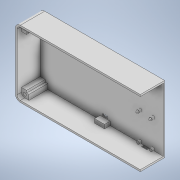
# Autodesk Inventor part: Case Left Half
Saved by Autodesk Inventor 2020 (Build 240168000, 168)
## iProperties
Created: 2021-04-14
Part Number: Case Left Half
Material: Generic
Document SubType Name: Modeling
Designer: user
Density: 1 g/cm^3
Appearance: Default
Author: user
Autodesk Inventor part; units mm, degrees
ref_plane "YZ Plane" through (0, 0, 0) normal (1, 0, 0) x (0, 1, 0)
ref_plane "XZ Plane" through (0, 0, 0) normal (0, 1, 0) x (-1, 0, 0)
ref_plane "XY Plane" through (0, 0, 0) normal (0, 0, 1) x (1, 0, 0)
sketch "Sketch1" plane through (0, 0, 0) normal (0, 0, 1) x (1, 0, 0)
  line L0 (5, 0) -> (336, 0)
  line L1 (341, 5) -> (341, 96)
  line L2 (336, 101) -> (5, 101)
  line L3 (0, 96) -> (0, 5)
  arc A0 (5, 101) -> (0, 96) centre (5, 96) ccw
  arc A1 (0, 5) -> (5, 0) centre (5, 5) ccw
  arc A2 (341, 96) -> (336, 101) centre (336, 96) ccw
  arc A3 (336, 0) -> (341, 5) centre (336, 5) ccw
  line L4 (5, 101.2) -> (336, 101.2)
  arc A4 (341.2, 96) -> (336, 101.2) centre (336, 96) ccw
  line L5 (341.2, 96) -> (341.2, 5)
  arc A5 (336, -0.2) -> (341.2, 5) centre (336, 5) ccw
  line L6 (336, -0.2) -> (5, -0.2)
  arc A6 (-0.2, 5) -> (5, -0.2) centre (5, 5) ccw
  line L7 (-0.2, 5) -> (-0.2, 96)
  arc A7 (5, 101.2) -> (-0.2, 96) centre (5, 96) ccw
  line L8 (5, 104) -> (336, 104)
  arc A8 (344, 96) -> (336, 104) centre (336, 96) ccw
  line L9 (344, 96) -> (344, 5)
  arc A9 (336, -3) -> (344, 5) centre (336, 5) ccw
  line L10 (336, -3) -> (5, -3)
  arc A10 (-3, 5) -> (5, -3) centre (5, 5) ccw
  line L11 (-3, 5) -> (-3, 96)
  arc A11 (5, 104) -> (-3, 96) centre (5, 96) ccw
  point P0 (0, 0)
  point P1 (341, 101)
  point P2 (0, 101)
  dimension "d0" = 341
  dimension "d1" = 101
  dimension "d2" = 5
  dimension "d3" = 0.2
  dimension "d4" = 3
  constraints: 24 end point, 24 point on circle, 12 centre point, 8 tangent, 6 parallel, 6 point on line, 3 equal radius, 3 perpendicular, 1 horizontal, 14 other
  measures "d0" distance of point (0, 101) point (341, 101)
  measures "d1" distance of point (0, 101) point (0, 0)
  measures "d2" radius of A0
  measures "d3" distance between parallel lines of L2 L4
  measures "d4" distance between parallel lines of L2 L8
extrude "Extrusion1" add sketch "Sketch1" along normal blind 2 contours A1 L3 A0 L2 A2 L1 A3 L0 | L4 A4 L5 A5 L6 A6 L7 A7 | L8 A8 L9 A9 L10 A10 L11 A11
sketch "Sketch2" plane through (0, 0, 2) normal (0, 0, 1) x (1, 0, 0)
  line L0 (5, 104) -> (336, 104)
  line L1 (344, 96) -> (344, 5)
  line L2 (336, -3) -> (5, -3)
  line L3 (-3, 5) -> (-3, 96)
  line L4 (344, 5) -> (344, 96) projected
  line L5 (5, -3) -> (336, -3) projected
  arc A0 (5, 104) -> (-3, 96) centre (5, 96) ccw
  arc A1 (-3, 5) -> (5, -3) centre (5, 5) ccw
  arc A2 (336, -3) -> (344, 5) centre (336, 5) ccw
  arc A3 (344, 96) -> (336, 104) centre (336, 96) ccw
  line L6 (336, 101.2) -> (5, 101.2)
  arc A4 (5, 101.2) -> (-0.2, 96) centre (5, 96) ccw
  line L7 (-0.2, 96) -> (-0.2, 5)
  arc A5 (-0.2, 5) -> (5, -0.2) centre (5, 5) ccw
  line L8 (5, -0.2) -> (336, -0.2)
  arc A6 (336, -0.2) -> (341.2, 5) centre (336, 5) ccw
  line L9 (341.2, 5) -> (341.2, 96)
  arc A7 (341.2, 96) -> (336, 101.2) centre (336, 96) ccw
  circle A8 centre (5, 96) radius 2.5
  line L10 (9, 92) -> (332, 92)
  line L11 (332, 92) -> (332, 9)
  line L12 (332, 9) -> (9, 9)
  line L13 (9, 9) -> (9, 92)
  line L14 (-0.2, 89.2) -> (8, 89.2)
  line L15 (8, 89.2) -> (8, 93)
  line L16 (8, 93) -> (11.8, 93)
  line L17 (11.8, 93) -> (11.8, 101.2)
  line L18 (9, 9) -> (332, 92)
  line L19 (170.5, 64.427) -> (170.5, 38.8649)
  line L20 (118.7328, 50.5) -> (212.1169, 50.5)
  circle A9 centre (336, 96) radius 2.5
  line L21 (341.2, 89.2) -> (333, 89.2)
  line L22 (333, 89.2) -> (333, 93)
  line L23 (333, 93) -> (329.2, 93)
  line L24 (329.2, 93) -> (329.2, 101.2)
  circle A10 centre (5, 5) radius 2.5
  line L25 (-0.2, 11.8) -> (8, 11.8)
  line L26 (8, 11.8) -> (8, 8)
  line L27 (8, 8) -> (11.8, 8)
  line L28 (11.8, 8) -> (11.8, -0.2)
  line L29 (329.2, 8) -> (329.2, -0.2)
  line L30 (333, 8) -> (329.2, 8)
  line L31 (333, 11.8) -> (333, 8)
  line L32 (341.2, 11.8) -> (333, 11.8)
  circle A11 centre (336, 5) radius 2.5
  point P0 (0, 0)
  dimension "d7" = 0
  dimension "d8" = 0
  dimension "d9" = 8
  dimension "d10" = 2.8
  dimension "d11" = 5
  dimension "d12" = 5.2
  dimension "d13" = 5.2
  dimension "d19" = 9.2
  dimension "d20" = 9.2
  dimension "d21" = 9.2
  dimension "d22" = 9.2
  dimension "d23" = 1
  dimension "d24" = 1
  dimension "d25" = 12
  dimension "d26" = 12
  constraints: 62 end point, 18 symmetric about line, 16 point on circle, 12 centre point, 8 tangent, 6 parallel, 6 perpendicular, 4 horizontal, 3 equal radius, 2 point on line, 1 vertical, 10 other
  measures "d7" distance between parallel lines of L1 L4
  measures "d8" distance between parallel lines of L2 L5
  measures "d9" radius of A0
  measures "d10" distance between parallel lines of L0 L6
  measures "d11" diameter of A8
  measures "d12" distance from line of A8.centre L6
  measures "d13" distance from line of A8.centre L7
  measures "d19" distance between parallel lines of L10 L6
  measures "d20" distance between parallel lines of L13 L7
  measures "d21" distance between parallel lines of L8 L12
  measures "d22" distance between parallel lines of L9 L11
  measures "d23" distance between parallel lines of L10 L16
  measures "d24" distance between parallel lines of L13 L15
  measures "d25" distance between parallel lines of L6 L14
  measures "d26" distance between parallel lines of L7 L17
extrude "Extrusion2" add sketch "Sketch2" along normal blind 30 contours L0 A3 L1 A2 L2 A1 L3 A0 | A7 L9 L21 L22 L23 L24 L6 | L17 L16 L15 L14 L7 A4 L6 | L9 A6 L8 L29 L30 L31 L32 | L25 L26 L27 L28 L8 A5 L7
sketch "Sketch3" plane through (0, 0, 32) normal (0, 0, 1) x (1, 0, 0)
  line L0 (5, 104) -> (336, 104)
  line L1 (344, 96) -> (344, 5)
  line L2 (336, -3) -> (5, -3)
  line L3 (-3, 5) -> (-3, 96)
  arc A0 (5, 104) -> (-3, 96) centre (5, 96) ccw
  arc A1 (-3, 5) -> (5, -3) centre (5, 5) ccw
  arc A2 (336, -3) -> (344, 5) centre (336, 5) ccw
  arc A3 (344, 96) -> (336, 104) centre (336, 96) ccw
  line L4 (336, 101.2) -> (5, 101.2)
  arc A4 (5, 101.2) -> (-0.2, 96) centre (5, 96) ccw
  line L5 (-0.2, 96) -> (-0.2, 5)
  arc A5 (-0.2, 5) -> (5, -0.2) centre (5, 5) ccw
  line L6 (5, -0.2) -> (336, -0.2)
  arc A6 (336, -0.2) -> (341.2, 5) centre (336, 5) ccw
  line L7 (341.2, 5) -> (341.2, 96)
  arc A7 (341.2, 96) -> (336, 101.2) centre (336, 96) ccw
  point P0 (0, 0)
  dimension "d29" = 8
  dimension "d30" = 2.8
  constraints: 16 end point, 16 point on circle, 8 centre point, 8 tangent, 4 parallel, 3 equal radius, 2 perpendicular, 1 horizontal, 7 other
  measures "d29" radius of A0
  measures "d30" distance between parallel lines of L0 L4
extrude "Extrusion3" add sketch "Sketch3" along normal blind 7
sketch "Sketch4" plane through (0, 0, 2) normal (0, 0, 1) x (1, 0, 0)
  line L0 (336, -0.2) -> (5, -0.2) projected
  line L1 (157.75, -0.2) -> (183.25, -0.2)
  line L2 (183.25, -0.2) -> (183.25, 48.2)
  line L3 (183.25, 48.2) -> (157.75, 48.2)
  line L4 (157.75, 48.2) -> (157.75, -0.2)
  line L5 (-0.2, 5) -> (-0.2, 96) projected
  circle A0 centre (160.25, 45.7) radius 2.3
  circle A1 centre (180.75, 45.7) radius 2.3
  circle A2 centre (160.25, 2.3) radius 2.3
  circle A3 centre (180.75, 2.3) radius 2.3
  point P0 (0, 0)
  dimension "d33" = 25.5
  dimension "d34" = 48.4
  dimension "d35" = 157.95
  dimension "d36" = 4.6
  dimension "d37" = 4.6
  dimension "d38" = 4.6
  dimension "d39" = 4.6
  dimension "d40" = 2.5
  dimension "d41" = 2.5
  dimension "d42" = 2.5
  dimension "d43" = 2.5
  dimension "d44" = 2.5
  dimension "d45" = 2.5
  dimension "d46" = 2.5
  dimension "d47" = 2.5
  constraints: 8 end point, 4 centre point, 2 parallel, 1 horizontal, 1 perpendicular, 1 point on line
  measures "d33" distance of L3.end L2.end
  measures "d34" distance of L2.end L1.end
  measures "d35" distance between parallel lines of L4 L5
  measures "d36" diameter of A0
  measures "d37" diameter of A1
  measures "d38" diameter of A2
  measures "d39" diameter of A3
  measures "d40" distance from line of L3 A0.centre
  measures "d41" distance from line of A0.centre L4
  measures "d42" distance from line of A1.centre L3
  measures "d43" distance from line of L2 A1.centre
  measures "d44" distance from line of L4 A2.centre
  measures "d45" distance from line of L1 A2.centre
  measures "d46" distance from line of L2 A3.centre
  measures "d47" distance from line of L1 A3.centre
extrude "Extrusion4" add sketch "Sketch4" along normal blind 4 contours A0 | A1 | A2 | A3
sketch "Sketch5" plane through (160.25, 2.3, 6) normal (0, 0, 1) x (1, 0, 0)
  circle A0 centre (0, 43.4) radius 2.3 projected
  circle A1 centre (0, 43.4) radius 1.5
  circle A2 centre (20.5, 43.4) radius 2.3 projected
  circle A3 centre (20.5, 43.4) radius 1.5
  circle A4 centre (0, 0) radius 2.3 projected
  circle A5 centre (0, 0) radius 1.5
  circle A6 centre (20.5, 0) radius 2.3 projected
  circle A7 centre (20.5, 0) radius 1.5
  point P0 (-160.25, -2.3)
  dimension "d50" = 3
  dimension "d51" = 3
  dimension "d52" = 3
  dimension "d53" = 3
  constraints: 4 centre point, 4 coincident
  measures "d50" diameter of A1
  measures "d51" diameter of A3
  measures "d52" diameter of A5
  measures "d53" diameter of A7
extrude "Extrusion5" add sketch "Sketch5" along normal blind 3 contours A1 | A3
chamfer "Chamfer1" distance 1 angle 45 2 edges at (158.75, 45.7, 9) (179.25, 45.7, 9)
sketch "Sketch6" plane through (5, -3, 0) normal (0, -1, 0) x (1, 0, 0)
  line L0 (161.3, 2.8) -> (169.7, 2.8)
  line L1 (169.7, 2.8) -> (169.7, 6.2)
  line L2 (169.7, 6.2) -> (161.3, 6.2)
  line L3 (161.3, 6.2) -> (161.3, 2.8)
  line L4 (6.8, 2) -> (324.2, 2) projected
  line L5 (0, 0) -> (0, 39) projected
  point P0 (-5, 0)
  dimension "d59" = 8.4
  dimension "d60" = 3.4
  dimension "d61" = 4.2
  dimension "d62" = 161.3
  constraints: 8 end point, 2 parallel, 1 horizontal, 1 perpendicular
  measures "d59" distance of L2.end L1.end
  measures "d60" distance of L0.end L1.end
  measures "d61" distance between parallel lines of L2 L4
  measures "d62" distance from line of L5 L2.end
extrude "Extrusion6" cut sketch "Sketch6" against normal blind 3
sketch "Sketch7" plane through (0, 0, 2) normal (0, 0, 1) x (1, 0, 0)
  line L0 (99.8, 7.8) -> (107.8, 7.8)
  line L1 (107.8, 7.8) -> (107.8, 10.8)
  line L2 (107.8, 10.8) -> (99.8, 10.8)
  line L3 (99.8, 10.8) -> (99.8, 7.8)
  line L4 (336, -0.2) -> (5, -0.2) projected
  line L5 (-0.2, 5) -> (-0.2, 96) projected
  point P0 (0, 0)
  dimension "d65" = 8
  dimension "d66" = 3
  dimension "d67" = 8
  dimension "d68" = 100
  constraints: 8 end point, 2 parallel, 1 horizontal, 1 perpendicular
  measures "d65" distance of L2.end L1.end
  measures "d66" distance of L1.end L0.end
  measures "d67" distance between parallel lines of L4 L0
  measures "d68" distance between parallel lines of L3 L5
extrude "Extrusion7" cut sketch "Sketch7" against normal blind 3
sketch "Sketch8" plane through (0, 0, 2) normal (0, 0, 1) x (1, 0, 0)
  line L0 (11.8, -0.2) -> (329.2, -0.2) projected
  line L1 (95.8, -0.2) -> (111.8, -0.2)
  line L2 (111.8, -0.2) -> (111.8, 5.95)
  line L3 (111.8, 5.95) -> (95.8, 5.95)
  line L4 (95.8, 5.95) -> (95.8, -0.2)
  line L5 (107.8, 7.8) -> (99.8, 7.8) projected
  line L6 (99.8, 7.8) -> (99.8, 10.8) projected
  point P0 (0, 0)
  dimension "d71" = 16
  dimension "d72" = 1.85
  dimension "d73" = 4
  constraints: 8 end point, 2 parallel, 1 horizontal, 1 perpendicular, 1 point on line
  measures "d71" distance of L3.end L2.end
  measures "d72" distance between parallel lines of L3 L5
  measures "d73" distance between parallel lines of L6 L4
extrude "Extrusion8" add sketch "Sketch8" along normal blind 9
sketch "Sketch9" plane through (0, 0, 39) normal (0, 0, 1) x (1, 0, 0)
  line L0 (-3, -16.474) -> (197, -16.474)
  line L1 (197, -16.474) -> (197, 116.8419)
  line L2 (197, 116.8419) -> (-3, 116.8419)
  line L3 (-3, 116.8419) -> (-3, -16.474)
  line L4 (-3, 96) -> (-3, 5) projected
  line L5 (197, 116.8419) -> (375.2281, 116.8419)
  line L6 (375.2281, 116.8419) -> (375.2281, -16.474)
  line L7 (375.2281, -16.474) -> (197, -16.474)
  line L8 (197, -16.474) -> (197, 116.8419)
  point P0 (0, 0)
  dimension "d76" = 200
  dimension "d77" = 0
  constraints: 16 end point, 4 parallel, 2 horizontal, 2 perpendicular
  measures "d76" distance of L1.end L2.end
  measures "d77" distance between parallel lines of L4 L3
extrude "Extrusion9" cut sketch "Sketch9" against normal blind 50 contours L1 L5 L6 L7
body "Solid1"
